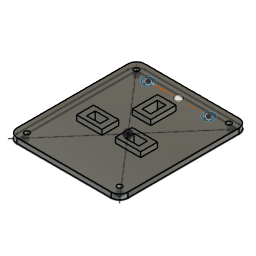
Upper_Layer v14 (Autodesk Fusion 360 design; units mm, degrees)
Autodesk Fusion 360 part; units mm, degrees
note: some values were not read from the file. Set by a fixed rule: which sketch regions a step uses.
sketch "Sketch1" plane through (0, 0, 0) normal (0, 0, 1) x (1, 0, 0) in component "Upper Layer"
  line L0 (30, -35) -> (-30, -35)
  line L1 (-30, -35) -> (-30, 35)
  line L2 (-30, 35) -> (30, 35)
  line L3 (30, 35) -> (30, -35)
  line L4 (30, -35) -> (-30, 35) construction
  line L5 (-30, -35) -> (30, 35) construction
  line L6 (28, -38) -> (-28, -38)
  line L7 (-33, -33) -> (-33, 33)
  line L8 (-28, 38) -> (28, 38)
  line L9 (33, 33) -> (33, -33)
  line L10 (33, -38) -> (-33, 38) construction
  line L11 (-33, -38) -> (33, 38) construction
  arc A0 (-28, 38) -> (-33, 33) centre (-28, 33) ccw
  arc A1 (33, 33) -> (28, 38) centre (28, 33) ccw
  arc A2 (-33, -33) -> (-28, -38) centre (-28, -33) ccw
  arc A3 (28, -38) -> (33, -33) centre (28, -33) ccw
  dimension "d1" = 60
  dimension "d2" = 70
  dimension "d3" = 66
  dimension "d4" = 76
  dimension "d51" = 5
  dimension "d52" = 5
  dimension "d53" = 5
  dimension "d54" = 5
  constraint horizontal L0
  constraint perpendicular L0 L1
  constraint parallel L0 L2
  constraint parallel L1 L3
  constraint coincident L4 origin
  constraint coincident L5 origin
  constraint horizontal L6
  constraint perpendicular L6 L7
  constraint parallel L6 L8
  constraint parallel L7 L9
  constraint coincident L10 origin
  constraint coincident L11 origin
  constraint coincident L10.end L7
  constraint coincident L10.end L8
  constraint tangent L7 A0
  constraint tangent L8 A0
  constraint coincident L11.end L8
  constraint coincident L11.end L9
  constraint tangent L8 A1
  constraint tangent L9 A1
  constraint coincident L11.start L7
  constraint coincident L11.start L6
  constraint tangent L7 A2
  constraint tangent L6 A2
  constraint coincident L10.start L9
  constraint coincident L10.start L6
  constraint tangent L9 A3
  constraint tangent L6 A3
  measures "d1" distance of L1.end L2.end
  measures "d2" distance of L0.end L1.end
  measures "d3" distance of L10.end L11.end
  measures "d4" distance of L11.start L10.end
  measures "d51" radius of A0
  measures "d52" radius of A1
  measures "d53" radius of A2
  measures "d54" radius of A3
extrude "Extrude1" add sketch "Sketch1" along normal blind 3 contours L0 L1 L2 L3 | L6 L7 L8 L9 A0 A1 A2 A3 in component "Upper Layer"
sketch "Sketch2" plane through (0, 0, 3) normal (0, 0, 1) x (-1, 0, 0) in component "Upper Layer"
  line L0 (-28, -38) -> (28, -38)
  line L1 (33, -33) -> (33, 33)
  line L2 (28, 38) -> (-28, 38)
  line L3 (-33, 33) -> (-33, -33)
  line L4 (-30, 35) -> (30, 35)
  line L5 (30, 35) -> (30, -35)
  line L6 (30, -35) -> (-30, -35)
  line L7 (-30, -35) -> (-30, 35)
  line L8 (-30, 35) -> (30, -35) construction
  line L9 (30, 35) -> (-30, -35) construction
  line L10 (0, 35) -> (0, -35) construction
  line L11 (2.5, -11) -> (-2.5, -11)
  line L12 (-2.5, -11) -> (-2.5, -20)
  line L13 (-2.5, -20) -> (2.5, -20)
  line L14 (2.5, -20) -> (2.5, -11)
  line L15 (2.5, -11) -> (-2.5, -20) construction
  line L16 (-2.5, -11) -> (2.5, -20) construction
  line L17 (0, -11) -> (0, 9) construction
  line L18 (0, 9) -> (-7.5, 9) construction
  line L19 (-7.5, 9) -> (-15.5, 9)
  line L20 (-15.5, 9) -> (-15.5, 4)
  line L21 (-15.5, 4) -> (-7.5, 4)
  line L22 (-7.5, 4) -> (-7.5, 9)
  line L23 (15.5, 4) -> (7.5, 4)
  line L24 (7.5, 4) -> (7.5, 9)
  line L25 (15.5, 9) -> (15.5, 4)
  line L26 (7.5, 9) -> (15.5, 9)
  line L27 (-5.5, -8) -> (5.5, -8)
  line L28 (5.5, -8) -> (5.5, -23)
  line L29 (5.5, -23) -> (-5.5, -23)
  line L30 (-5.5, -23) -> (-5.5, -8)
  line L31 (-5.5, -8) -> (5.5, -23) construction
  line L32 (5.5, -8) -> (-5.5, -23) construction
  line L33 (-11.5, 9) -> (-11.5, 4) construction
  line L34 (-7.5, 6.5) -> (-15.5, 6.5) construction
  line L35 (-19, 11.5) -> (-4, 11.5)
  line L36 (-4, 11.5) -> (-4, 1.5)
  line L37 (-4, 1.5) -> (-19, 1.5)
  line L38 (-19, 1.5) -> (-19, 11.5)
  line L39 (-19, 11.5) -> (-4, 1.5) construction
  line L40 (-4, 11.5) -> (-19, 1.5) construction
  line L41 (4, 1.5) -> (19, 1.5)
  line L42 (4, 11.5) -> (4, 1.5)
  line L43 (19, 11.5) -> (4, 11.5)
  line L44 (19, 1.5) -> (19, 11.5)
  arc A0 (33, 33) -> (28, 38) centre (28, 33) ccw
  arc A1 (-28, 38) -> (-33, 33) centre (-28, 33) ccw
  arc A2 (-33, -33) -> (-28, -38) centre (-28, -33) ccw
  arc A3 (28, -38) -> (33, -33) centre (28, -33) ccw
  point P0 (0, -15.5)
  point P1 (0, -15.5)
  point P2 (-11.5, 6.5)
  dimension "d7" = 5
  dimension "d8" = 9
  dimension "d9" = 20
  dimension "d10" = 7.5
  dimension "d11" = 8
  dimension "d12" = 5
  dimension "d13" = 11
  dimension "d14" = 15
  dimension "d15" = 15
  dimension "d16" = 10
  constraint horizontal L4
  constraint perpendicular L4 L5
  constraint parallel L4 L6
  constraint parallel L5 L7
  constraint coincident L8 origin
  constraint coincident L9 origin
  constraint midpoint L4 L10.start
  constraint midpoint L6 L10.end
  constraint horizontal L11
  constraint perpendicular L11 L12
  constraint parallel L11 L13
  constraint parallel L12 L14
  constraint coincident L15 P1
  constraint coincident L16 P1
  constraint coincident L10 P1
  constraint midpoint L11 L17.start
  constraint perpendicular L11 L17
  constraint perpendicular L17 L18
  constraint horizontal L19
  constraint vertical L20
  constraint horizontal L21
  constraint vertical L22
  constraint symmetric L10 L18.end L24.end
  constraint symmetric L10 L19.end L25.start
  constraint symmetric L10 L20.end L23.start
  constraint symmetric L10 L21.end L23.end
  constraint horizontal L27
  constraint perpendicular L27 L28
  constraint parallel L27 L29
  constraint parallel L28 L30
  constraint coincident L31 P1
  constraint coincident L32 P1
  constraint coincident P1 P0
  constraint midpoint L19 L33.start
  constraint midpoint L21 L33.end
  constraint midpoint L22 L34.start
  constraint midpoint L20 L34.end
  constraint horizontal L35
  constraint perpendicular L35 L36
  constraint parallel L35 L37
  constraint parallel L36 L38
  constraint coincident L39 P2
  constraint coincident L40 P2
  constraint midpoint L33 P2
  constraint symmetric L10 L35.start L43.start
  constraint symmetric L10 L35.end L42.start
  constraint symmetric L10 L36.end L41.start
  constraint symmetric L10 L37.end L41.end
  measures "d7" distance of L12.end L13.end
  measures "d8" distance of L11.end L12.end
  measures "d9" distance of L17.start L17.end
  measures "d10" distance of L17.end L18.end
  measures "d11" distance of L18.end L19.end
  measures "d12" distance of L18.end L21.end
  measures "d13" distance of L28.end L29.end
  measures "d14" distance of L27.end L28.end
  measures "d15" distance of L36.end L37.end
  measures "d16" distance of L35.end L36.end
extrude "Extrude2" cut sketch "Sketch2" against normal up to surface (3 mm away) contours L11 L12 L13 L14 in component "Upper Layer"
extrude "Extrude3" add sketch "Sketch2" along normal blind 3 contours L27 L28 L29 L30 in component "Upper Layer"
extrude "Extrude4" cut sketch "Sketch2" against normal up to surface (3 mm away) contours L19 L20 L21 L22 | L23 L24 L25 L26 in component "Upper Layer"
extrude "Extrude5" add sketch "Sketch2" along normal blind 3 contours L35 L36 L37 L38 | L41 L42 L43 L44 in component "Upper Layer"
sketch "Sketch2 (2)" plane through (0, 0, -8.9199) normal (0, 0, -1) x (1, 0, 0)
  line L0 (22.45, -32.5) -> (22.45, -27.6)
  line L1 (22.45, -27.6) -> (17.55, -27.6)
  line L2 (17.55, -27.6) -> (17.55, -32.5)
  line L3 (17.55, -32.5) -> (22.45, -32.5)
  line L4 (-17.55, -32.45) -> (-17.55, -27.55)
  line L5 (-17.55, -27.55) -> (-22.45, -27.55)
  line L6 (-22.45, -27.55) -> (-22.45, -32.45)
  line L7 (-22.45, -32.45) -> (-17.55, -32.45)
sketch "Sketch4" plane through (0, 0, 3) normal (0, 0, 1) x (1, 0, 0) in component "Upper Layer"
  line L0 (0, 30) -> (-18, 30) construction
  circle A0 centre (-18, 30) radius 3
  line L1 (-18, 30) -> (-15, 30)
  line L2 (-18, 30) -> (-7.5877, 30) construction
  line L3 (-18, 30) -> (18, 30) construction
  circle A1 centre (18, 30) radius 3
  dimension "d37" = 6
  dimension "d38" = 36
  dimension "d39" = 6
  dimension "d50" = 18
  constraint horizontal L0
  constraint coincident L0.end A0.centre
  constraint coincident A0 L1.end
  constraint coincident L0 L1.end
  constraint coincident L0 L2.end
  constraint parallel L1 L3
  constraint coincident L3.end A1.centre
  measures "d37" diameter of A0
  measures "d38" distance of L0.end L3.end
  measures "d39" diameter of A1
  measures "d50" distance of L0.start L0.end
extrude "Extrude9" cut sketch "Sketch4" against normal up to surface (3 mm away) in component "Upper Layer"
sketch "Sketch3" plane through (0, 0, 3) normal (0, 0, 1) x (-1, 0, 0)
  line L0 (30, 35) -> (27.5, 35) construction
  line L1 (30, 35) -> (30, 32.5) construction
  circle A0 centre (27.5, 32.5) radius 2.5
  line L2 (40, 0) -> (-40, 0)
  line L3 (0, -45) -> (0, 47.452)
  circle A1 centre (27.5, -32.5) radius 2.5
  circle A2 centre (-27.5, -32.5) radius 2.5
  circle A3 centre (-27.5, 32.5) radius 2.5
  circle A4 centre (27.5, -32.5) radius 1.5
  circle A5 centre (27.5, 32.5) radius 1.5
  circle A6 centre (-27.5, -32.5) radius 1.5
  circle A7 centre (-27.5, 32.5) radius 1.5
  dimension "d42" = 2.5
  dimension "d43" = 2.5
  dimension "d44" = 3
  dimension "d45" = 3
  dimension "d46" = 3
  dimension "d47" = 3
  constraint horizontal L0
  constraint perpendicular L0 L1
  constraint coincident L0.end A0
  constraint coincident L1.end A0
  constraint tangent L1 A0
  constraint tangent L0 A0
  constraint horizontal L2
  constraint vertical L3
  constraint symmetric A0 L2 A1
  constraint symmetric A0 L3 A3
  constraint symmetric L3 A1 A2
  constraint concentric A1 A4
  constraint concentric A0 A5
  constraint concentric A2 A6
  constraint concentric A3 A7
  measures "d42" distance of L0.start L0.end
  measures "d43" distance of L0.start L1.end
  measures "d44" diameter of A4
  measures "d45" diameter of A5
  measures "d46" diameter of A6
  measures "d47" diameter of A7
extrude "Extrude10" cut sketch "Sketch3" against normal blind 3 contours A4 | A5 | A6 | A7 in component "Upper Layer"
component "Upper Layer" placed x (1, 0, 0) y (0, 1, 0) z (0, 0, 1) at (0, 0, 0)
equation "d10 = ( 15 / 2 ) * 1 mm"
